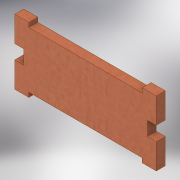
# Autodesk Inventor part: boxFront
Saved by Autodesk Inventor 2017 (Build 210142000, 142)
## iProperties
Created: 2017-05-22
Part Number: boxFront
Material: Generic
Document SubType Name: Modeling
Designer: Dominic Gaiero
Density: 1 g/cm^3
Appearance: Walnut - Natural Polished
Author: Dominic Gaiero
Autodesk Inventor part; units mm, degrees
ref_plane "YZ Plane" through (0, 0, 0) normal (1, 0, 0) x (0, 1, 0)
ref_plane "XZ Plane" through (0, 0, 0) normal (0, 1, 0) x (-1, 0, 0)
ref_plane "XY Plane" through (0, 0, 0) normal (0, 0, 1) x (1, 0, 0)
sketch "Sketch1" plane through (0, 0, 0) normal (0, 0, 1) x (1, 0, 0)
  line L0 (349.5941, 169.6239) -> (430.3941, 169.6239)
  line L1 (430.3941, 209.6239) -> (349.5941, 209.6239)
  line L2 (349.5941, 209.6239) -> (349.5941, 212.7989)
  line L3 (349.5941, 212.7989) -> (339.5941, 212.7989)
  line L4 (339.5941, 212.7989) -> (339.5941, 212.7989)
  line L5 (430.3941, 209.6239) -> (430.3941, 212.7989)
  line L6 (430.3941, 212.7989) -> (440.3941, 212.7989)
  line L7 (440.3941, 212.7989) -> (440.3941, 212.7989)
  line L8 (349.5941, 169.6239) -> (349.5941, 166.4489)
  line L9 (349.5941, 166.4489) -> (339.5941, 166.4489)
  line L10 (339.5941, 166.4489) -> (339.5941, 172.7989)
  line L11 (430.3941, 169.6239) -> (430.3941, 166.4489)
  line L12 (430.3941, 166.4489) -> (440.3941, 166.4489)
  line L13 (440.3941, 166.4489) -> (440.3941, 172.7989)
  line L14 (339.5941, 194.6239) -> (345.9441, 194.6239)
  line L15 (345.9441, 194.6239) -> (345.9441, 184.6239)
  line L16 (345.9441, 184.6239) -> (339.5941, 184.6239)
  line L17 (440.3941, 194.6239) -> (434.0441, 194.6239)
  line L18 (434.0441, 194.6239) -> (434.0441, 184.6239)
  line L19 (434.0441, 184.6239) -> (440.3941, 184.6239)
  line L20 (440.3941, 172.7989) -> (440.3941, 184.6239)
  line L21 (440.3941, 194.6239) -> (440.3941, 212.7989)
  line L22 (339.5941, 212.7989) -> (339.5941, 194.6239)
  line L23 (339.5941, 184.6239) -> (339.5941, 172.7989)
  line L24 (389.9941, 209.6239) -> (389.9941, 169.6239)
  point P0 (0, 0)
  point P1 (339.5941, 192.7989)
  point P2 (339.5941, 192.7989)
  point P3 (345.9441, 189.6239)
  point P4 (389.9941, 189.6239)
  point P5 (434.0441, 189.6239)
  dimension "d16" = 6.35
  dimension "d0" = 40
  dimension "d1" = 100.8
  dimension "d2" = 10
  dimension "d3" = 6.35
  dimension "d4" = 6.35
  dimension "d5" = 10
  dimension "d6" = 10
  dimension "d7" = 10
  dimension "d8" = 10
  dimension "d9" = 3.175
  dimension "d10" = 3.175
  dimension "d11" = 3.175
  dimension "d12" = 3.175
  dimension "d13" = 10
  dimension "d14" = 6.35
  dimension "d15" = 6.35
  constraints: 50 end point, 11 parallel, 5 midpoint, 4 perpendicular, 3 horizontal, 2 horizontal alignment, 1 coincident
  measures "d0" distance between parallel lines of L0 L1
  measures "d1" distance between parallel lines of L22 L21
  measures "d2" distance between parallel lines of L16 L14
  measures "d3" distance between parallel lines of L22 L15
  measures "d4" distance between parallel lines of L21 L18
  measures "d5" distance between parallel lines of L4 L2
  measures "d6" distance between parallel lines of L7 L5
  measures "d7" distance between parallel lines of L13 L11
  measures "d8" distance between parallel lines of L10 L8
  measures "d9" distance between parallel lines of L0 L9
  measures "d10" distance between parallel lines of L1 L3
  measures "d11" distance between parallel lines of L1 L6
  measures "d12" distance between parallel lines of L0 L12
  measures "d13" distance between parallel lines of L19 L17
  measures "d14" distance of L18.end L19.end
  measures "d15" distance of L15.end L16.end
extrude "Extrusion1" add sketch "Sketch1" along normal blind 6.35
body "Solid1"
